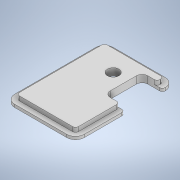
# Autodesk Inventor part: proxima_cup
Saved by Autodesk Inventor 2021 (Build 250183000, 183)
## iProperties
Created: 2022-01-29
Part Number: proxima_cup
Material: Generic
Document SubType Name: Modeling
Designer: ermoz
Density: 1 g/cm^3
Appearance: Default
Author: ermoz
Autodesk Inventor part; units mm, degrees
ref_plane "YZ Plane" through (0, 0, 0) normal (1, 0, 0) x (0, 1, 0)
ref_plane "XZ Plane" through (0, 0, 0) normal (0, 1, 0) x (-1, 0, 0)
ref_plane "XY Plane" through (0, 0, 0) normal (0, 0, 1) x (1, 0, 0)
sketch "Sketch1" plane through (0, 0, 0) normal (0, 1, 0) x (-1, 0, 0)
  line L0 (-6, 8.5) -> (6, 8.5)
  line L1 (6, 8.5) -> (6, -8.5)
  line L2 (6, -8.5) -> (-6, -8.5)
  line L3 (-6, -8.5) -> (-6, 8.5)
  line L4 (-6, 8.5) -> (6, -8.5) construction
  line L5 (6, 8.5) -> (-6, -8.5) construction
  point P0 (0, 0)
  dimension "d0" = 12
  dimension "d1" = 17
  constraints: 12 end point, 2 midpoint, 2 parallel, 1 horizontal, 1 perpendicular
  measures "d0" distance of L0.start L0.end
  measures "d1" distance of L0.end L1.end
extrude "Extrusion1" add sketch "Sketch1" along normal blind 0.5
sketch "Sketch2" plane through (0, 0.5, 0) normal (0, 1, 0) x (1, 0, 0)
  line L0 (5.1, -7.6) -> (-5.1, -7.6)
  line L1 (-5.1, -7.6) -> (-5.1, 7.6)
  line L2 (-5.1, 7.6) -> (5.1, 7.6)
  line L3 (5.1, 7.6) -> (5.1, -7.6)
  line L4 (5.1, -7.6) -> (-5.1, 7.6) construction
  line L5 (-5.1, -7.6) -> (5.1, 7.6) construction
  point P0 (0, 0)
  dimension "d4" = 15.2
  dimension "d5" = 10.2
  constraints: 12 end point, 2 midpoint, 2 parallel, 1 horizontal, 1 perpendicular
  measures "d4" distance of L0.end L1.end
  measures "d5" distance of L1.end L2.end
extrude "Extrusion2" add sketch "Sketch2" along normal blind 0.75
fillet "Fillet1" radius 1.5 4 edges at (-6, 0.25, 8.5) (6, 0.25, 8.5) (6, 0.25, -8.5) (-6, 0.25, -8.5)
fillet "Fillet2" radius 0.5 4 edges at (5.1, 0.875, -7.6) (-5.1, 0.875, -7.6) (-5.1, 0.875, 7.6) (5.1, 0.875, 7.6)
sketch "Sketch3" plane through (0, 0, 0) normal (0, -1, 0) x (1, 0, 0)
  line L0 (5, 0) -> (3.5, 0)
  line L1 (2.5, -1) -> (2.5, -5.5)
  line L2 (3.5, -6.5) -> (5, -6.5)
  line L3 (5, -6.5) -> (5, 0)
  line L4 (5, 0) -> (8.5853, 0)
  line L5 (8.5853, 0) -> (8.5853, -6.5)
  line L6 (8.5853, -6.5) -> (5, -6.5)
  line L7 (5, -6.5) -> (5, 0)
  line L8 (4.5, -8.5) -> (-4.5, -8.5) projected
  line L9 (6, 7) -> (6, -7) projected
  circle A0 centre (0, -4) radius 1
  line L10 (-6, -7) -> (-6, 7) projected
  arc A1 (3.5, 0) -> (2.5, -1) centre (3.5, -1) ccw
  arc A2 (2.5, -5.5) -> (3.5, -6.5) centre (3.5, -5.5) ccw
  point P0 (0, 0)
  point P1 (2.5, -6.5)
  point P2 (6, -6.5)
  point P3 (6, 0)
  dimension "d10" = 6.5
  dimension "d11" = 2.5
  dimension "d12" = 2
  dimension "d13" = 3.5
  dimension "d14" = 6
  dimension "d15" = 4.5
  dimension "d16" = 2
  dimension "d17" = 1
  constraints: 16 end point, 4 parallel, 4 point on circle, 4 tangent, 3 centre point, 3 point on line, 2 horizontal, 2 perpendicular, 1 equal radius
  measures "d10" distance of L2.end L0.start
  measures "d11" distance of point (2.5, -6.5) L2.end
  measures "d12" distance between parallel lines of L8 L2
  measures "d13" distance between parallel lines of L9 L1
  measures "d14" distance from line of L10 A0.centre
  measures "d15" distance from line of L8 A0.centre
  measures "d16" diameter of A0
  measures "d17" radius of A1
extrude "Extrusion3" cut sketch "Sketch3" against normal up to surface (1.25 mm away) contours L3 L2 A2 L1 A1 L0 | L4 L9 L6 L3 | A0
fillet "Fillet3" radius 0.5 4 edges at (5.1, 0.875, 0) (5.1, 0.875, -6.5) (6, 0.25, -6.5) (6, 0.25, 0)
body "Solid1"
